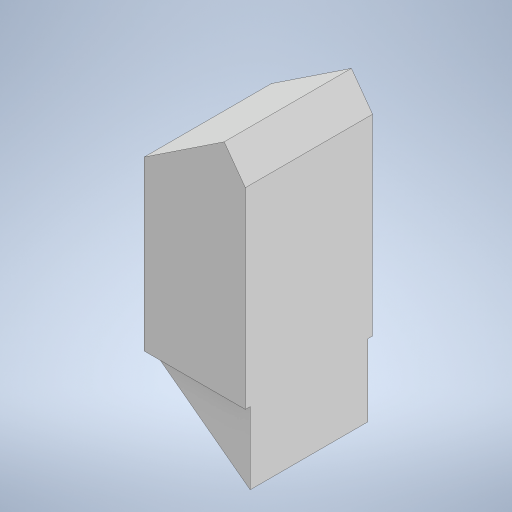
# Autodesk Inventor part: 頭 小小屋
Saved by Autodesk Inventor 2024 (Build 280153000, 153)
## iProperties
Created: 2024-05-23
Part Number: 頭 小小屋
Material: 一般
Document SubType Name: Modeling
Designer: User
Density: 1 g/cm^3
Appearance: 預設
Author: User
Autodesk Inventor part; units mm, degrees
ref_plane "YZ Plane" through (0, 0, 0) normal (1, 0, 0) x (0, 1, 0)
ref_plane "XZ Plane" through (0, 0, 0) normal (0, 1, 0) x (-1, 0, 0)
ref_plane "XY Plane" through (0, 0, 0) normal (0, 0, 1) x (1, 0, 0)
sketch "草圖1" plane through (0, 0, 0) normal (0, 0, 1) x (1, 0, 0)
  line L0 (0, 0) -> (0, 7)
  line L1 (0, 7) -> (3.3317, 9.2136)
  line L2 (3.3317, 9.2136) -> (4.2133, 8)
  line L3 (4.2133, 8) -> (4.2133, 0)
  line L4 (4.2133, 0) -> (0, 0)
  dimension "d0" = 7
  dimension "d1" = 4
  dimension "d2" = 1.5
  dimension "d3" = 8
  constraints: 10 end point, 1 parallel, 1 perpendicular, 1 vertical
  measures "d0" distance of L0.start L0.end
  measures "d1" distance of L0.end L1.end
  measures "d2" distance of L1.end L2.end
  measures "d3" distance of L2.end L3.end
extrude "擠出1" add sketch "草圖1" along normal blind 5.3
sketch "草圖2" plane through (0, 0, 0) normal (-1, 0, 0) x (0, 0, 1)
  line L0 (1, 2.25) -> (4.3, 2.25)
  line L1 (4.4, 2.35) -> (4.4, 5.65)
  line L2 (4.3, 5.75) -> (1, 5.75)
  line L3 (0.9, 5.65) -> (0.9, 2.35)
  line L4 (0.9, 2.25) -> (4.4, 5.75) construction
  line L5 (4.4, 2.25) -> (0.9, 5.75) construction
  line L6 (1.2, 5.55) -> (2.2, 5.55)
  line L7 (2.3, 5.45) -> (2.3, 4.45)
  line L8 (2.2, 4.35) -> (1.2, 4.35)
  line L9 (1.1, 4.45) -> (1.1, 5.45)
  line L10 (1.1, 5.55) -> (2.3, 4.35) construction
  line L11 (2.3, 5.55) -> (1.1, 4.35) construction
  line L12 (3.1, 4.35) -> (4.1, 4.35)
  line L13 (4.2, 4.45) -> (4.2, 5.45)
  line L14 (4.1, 5.55) -> (3.1, 5.55)
  line L15 (3, 5.45) -> (3, 4.45)
  line L16 (3, 4.35) -> (4.2, 5.55) construction
  line L17 (4.2, 4.35) -> (3, 5.55) construction
  line L18 (3.1, 3.65) -> (4.1, 3.65)
  line L19 (4.2, 3.55) -> (4.2, 2.55)
  line L20 (4.1, 2.45) -> (3.1, 2.45)
  line L21 (3, 2.55) -> (3, 3.55)
  line L22 (3, 3.65) -> (4.2, 2.45) construction
  line L23 (4.2, 3.65) -> (3, 2.45) construction
  line L24 (1.2, 2.45) -> (2.2, 2.45)
  line L25 (2.3, 2.55) -> (2.3, 3.55)
  line L26 (2.2, 3.65) -> (1.2, 3.65)
  line L27 (1.1, 3.55) -> (1.1, 2.55)
  line L28 (1.1, 2.45) -> (2.3, 3.65) construction
  line L29 (2.3, 2.45) -> (1.1, 3.65) construction
  arc A0 (1, 5.75) -> (0.9, 5.65) centre (1, 5.65) ccw
  arc A1 (0.9, 2.35) -> (1, 2.25) centre (1, 2.35) ccw
  arc A2 (4.3, 2.25) -> (4.4, 2.35) centre (4.3, 2.35) ccw
  arc A3 (4.4, 5.65) -> (4.3, 5.75) centre (4.3, 5.65) ccw
  arc A4 (4.2, 5.45) -> (4.1, 5.55) centre (4.1, 5.45) ccw
  arc A5 (4.1, 4.35) -> (4.2, 4.45) centre (4.1, 4.45) ccw
  arc A6 (3, 4.45) -> (3.1, 4.35) centre (3.1, 4.45) ccw
  arc A7 (3.1, 5.55) -> (3, 5.45) centre (3.1, 5.45) ccw
  arc A8 (2.3, 5.45) -> (2.2, 5.55) centre (2.2, 5.45) ccw
  arc A9 (1.2, 5.55) -> (1.1, 5.45) centre (1.2, 5.45) ccw
  arc A10 (1.1, 4.45) -> (1.2, 4.35) centre (1.2, 4.45) ccw
  arc A11 (2.2, 4.35) -> (2.3, 4.45) centre (2.2, 4.45) ccw
  arc A12 (2.3, 3.55) -> (2.2, 3.65) centre (2.2, 3.55) ccw
  arc A13 (2.2, 2.45) -> (2.3, 2.55) centre (2.2, 2.55) ccw
  arc A14 (1.1, 2.55) -> (1.2, 2.45) centre (1.2, 2.55) ccw
  arc A15 (1.2, 3.65) -> (1.1, 3.55) centre (1.2, 3.55) ccw
  arc A16 (3.1, 3.65) -> (3, 3.55) centre (3.1, 3.55) ccw
  arc A17 (4.2, 3.55) -> (4.1, 3.65) centre (4.1, 3.55) ccw
  arc A18 (4.1, 2.45) -> (4.2, 2.55) centre (4.1, 2.55) ccw
  arc A19 (3, 2.55) -> (3.1, 2.45) centre (3.1, 2.55) ccw
  point P0 (2.65, 4)
  point P1 (1.7, 4.95)
  point P2 (3.6, 4.95)
  point P3 (3.6, 3.05)
  point P4 (1.7, 3.05)
  dimension "d7" = 3.5
  dimension "d8" = 3.5
  dimension "d9" = 1.2
  dimension "d10" = 1.2
  dimension "d11" = 0.2
  dimension "d12" = 0.1
  dimension "d13" = 0.1
  constraints: 60 end point, 49 point on line, 40 point on circle, 40 tangent, 20 centre point, 18 equal radius, 10 midpoint, 10 parallel, 5 horizontal, 5 perpendicular
  measures "d7" distance of L5.end L4.end
  measures "d8" distance of L4.end L5.start
  measures "d9" distance of L10.end L11.end
  measures "d10" distance of L11.start L10.end
  measures "d11" distance between parallel lines of L2 L6
  measures "d12" radius of A0
  measures "d13" radius of A4
extrude "擠出2" add sketch "草圖2" along normal blind 0.2
extrude "擠出3" cut sketch "草圖2" against normal blind 0.1 contours L6 A8 L7 A11 L8 A10 L9 A9 | A6 L15 A7 L14 A4 L13 A5 L12 | L18 A17 L19 A18 L20 A19 L21 A16 | A14 L27 A15 L26 A12 L25 A13 L24
sketch "草圖3" plane through (0, 0, 0) normal (0, -1, 0) x (1, 0, 0)
  line L0 (4.2133, 0) -> (4.2133, 5.3) projected
  line L1 (4.2133, 0.2) -> (0.2, 0.2)
  line L2 (0.2, 0.2) -> (0.2, 5.1)
  line L3 (0.2, 5.1) -> (4.2133, 5.1)
  line L4 (4.2133, 5.1) -> (4.2133, 0.2)
  line L5 (0, 0) -> (4.2133, 0) projected
  line L6 (0, 0) -> (0, 5.3) projected
  line L7 (0, 5.3) -> (4.2133, 5.3) projected
  dimension "d18" = 0.2
  dimension "d19" = 0.2
  dimension "d20" = 0.2
  constraints: 8 end point, 2 parallel, 1 horizontal, 1 perpendicular, 1 point on line
  measures "d18" distance between parallel lines of L5 L1
  measures "d19" distance between parallel lines of L6 L2
  measures "d20" distance between parallel lines of L7 L3
extrude "擠出4" add sketch "草圖3" along normal blind 3 contours L1 L2 L3 L0
sketch "草圖4" plane through (0.2, 0, 5.1) normal (0, 0, 1) x (1, 0, 0)
  line L0 (4.0133, 0) -> (0, 0) projected
  line L1 (0, 0) -> (4.0133, -3)
  line L2 (0, -3) -> (4.0133, -3) projected
  line L3 (4.0133, -3) -> (0, -3)
  line L4 (0, -3) -> (0, 0)
  point P0 (-0.2, 0)
  constraints: 6 end point, 1 collinear, 1 perpendicular
extrude "擠出5" cut sketch "草圖4" against normal up to surface (4.9 mm away)
